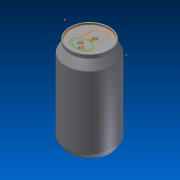
# Autodesk Inventor part: cocacola can
Saved by Autodesk Inventor 2019 (Build 230136000, 136)
## iProperties
Created: 2011-12-12
Part Number: cocacola can
Material: Generic
Document SubType Name: Modeling
Designer: roedger3
Density: 1 g/cm^3
Appearance: Default
Author: roedger3
Autodesk Inventor part; units mm, degrees
ref_plane "YZ Plane" through (0, 0, 0) normal (1, 0, 0) x (0, 1, 0)
ref_plane "XZ Plane" through (0, 0, 0) normal (0, 1, 0) x (-1, 0, 0)
ref_plane "XY Plane" through (0, 0, 0) normal (0, 0, 1) x (1, 0, 0)
sketch "Sketch1" plane through (0, 0, 0) normal (0, 0, 1) x (1, 0, 0)
  line L0 (-5.0988, -3.9037) -> (-5.0988, -101.0858)
  line L1 (0.463, -109.3372) -> (-0.635, -109.3372)
  line L2 (1.0329, 8.8525) -> (1.0329, 10.9702)
  line L3 (0.6383, 7.3196) -> (-4.7042, -2.3707)
  line L4 (-0.635, -109.3372) -> (-0.635, -109.3228)
  line L5 (-1.2355, -107.4647) -> (-4.4983, -102.9439)
  arc A0 (-5.0988, -101.0858) -> (-4.4983, -102.9439) centre (-1.9238, -101.0858) ccw
  arc A1 (-0.635, -109.3228) -> (-1.2355, -107.4647) centre (-3.81, -109.3228) ccw
  arc A2 (-4.7042, -2.3707) -> (-5.0988, -3.9037) centre (-1.9238, -3.9037) ccw
  arc A3 (0.6383, 7.3196) -> (1.0329, 8.8525) centre (-2.1421, 8.8525) ccw
  line L6 (1.0329, 10.9702) -> (0.6426, 10.9702)
  line L7 (0.3886, 11.2242) -> (0.3886, 13.0908)
  line L8 (0.6426, 13.3448) -> (1.5362, 13.3448)
  line L9 (1.7902, 13.0908) -> (1.7902, 11.2242)
  line L10 (2.0442, 10.9702) -> (27.7942, 10.9702)
  arc A4 (0.3886, 11.2242) -> (0.6426, 10.9702) centre (0.6426, 11.2242) ccw
  arc A5 (0.6426, 13.3448) -> (0.3886, 13.0908) centre (0.6426, 13.0908) ccw
  arc A6 (1.7902, 13.0908) -> (1.5362, 13.3448) centre (1.5362, 13.0908) ccw
  arc A7 (1.7902, 11.2242) -> (2.0442, 10.9702) centre (2.0442, 11.2242) ccw
  line L11 (27.7942, 10.9702) -> (27.7942, -95.2167)
  ellipse E0 centre (27.7942, 0) end of major axis (-3.3972, 0) minor radius 9.4787 (27.7942, 9.4787) -> (2.7229, 5.6391) ccw
  arc A8 (2.7229, 5.6391) -> (-4.9986, -3.1122) centre (11.6697, -10.0371) ccw
  arc A9 (27.7942, -95.2167) -> (3.1136, -106.0246) centre (27.585, -128.3229) ccw
  ellipse E1 centre (27.7942, -109.3372) end of major axis (27.7942, -101.6264) minor radius 27.3312 (27.7942, -101.6264) -> (0.463, -109.3372) ccw
  line L12 (27.7942, -95.2167) -> (27.7942, -101.6264)
  point P0 (0, 0)
  dimension "d8" = 3.175
  dimension "d20" = 0.254
  dimension "d21" = 122.682
  constraints: 26 end point, 21 point on circle, 15 tangent, 10 centre point, 6 equal radius, 4 perpendicular, 2 point on line, 2 vertical, 1 horizontal, 1 parallel, 9 other
  measures "d8" radius of A0
  measures "d20" radius of A4
  measures "d21" distance from line of L1 L8.start
revolve "Revolution1" add sketch "Sketch1" angle 360 about axis through (27.7942, 10.9702, 0) along (0, -1, 0) contours A2 A8 L3 E0 L11 A9 E1 L1 L4 A1 L5 A0 L0 | A2 L3 A8 | L3 A3 L2 L6 A4 L7 A5 L8 A6 L9 A7 L10 L11 E0 A8
sketch "Sketch3" plane through (27.7942, 10.9702, 0) normal (0, 1, 0) x (1, 0, 0)
  circle A0 centre (0, 0) radius 25.75 projected
  point P0 (-27.7942, 0)
sketch "Sketch4" plane through (27.7942, 10.9702, 0) normal (0, 1, 0) x (1, 0, 0)
  ellipse E0 centre (-0.043, -10.033) end of major axis (-11.981, -10.033) minor radius 8.255
  point P0 (-27.7942, 0)
  dimension "d23" = 11.938
  dimension "d24" = 8.255
  constraints: 2 other
sketch "Sketch5" plane through (27.7942, 10.9702, 0) normal (0, 1, 0) x (1, 0, 0)
  circle A0 centre (0, 0) radius 25.75 projected
  point P0 (-27.7942, 0)
shell "Shell1" [suppressed]
sketch "Sketch6" plane through (27.7942, 10.9702, 0) normal (0, 1, 0) x (1, 0, 0)
  ellipse E0 centre (-0.043, -10.033) end of major axis (11.895, -10.033) minor radius 8.255 projected
  circle A0 centre (0, 0) radius 25.75 projected
  ellipse E1 centre (-0.043, -10.033) end of major axis (-0.043, 0) minor radius 13.716 (-11.748, -4.803) -> (11.6621, -4.803) ccw
  arc A1 (9.3327, 9.75) -> (-9.3977, 9.637) centre (-0.043, 11.4301) ccw
  line L0 (0, 0) -> (0, 1.9052)
  arc A2 (-11.748, -4.803) -> (-9.568, 11.4301) centre (-41.662, 7.4773) ccw
  arc A3 (9.482, 11.4301) -> (11.6621, -4.803) centre (42.7111, 7.6297) ccw
  point P0 (-27.7942, 0)
  dimension "d8" = 3.175
  dimension "d33" = 13.716
  dimension "d34" = 10.033
  constraints: 11 point on circle, 3 centre point, 2 end point, 1 coincident, 1 vertical, 5 other
extrude "Extrusion2" cut sketch "Sketch6" against normal blind 0.254 contours A2 A1 A3 E1
sketch "Sketch7" plane through (27.7942, 10.7162, 0) normal (0, 1, 0) x (1, 0, 0)
  circle A0 centre (0, 0) radius 1.905
  point P0 (11.895, -10.033)
  point P1 (-27.7942, 0)
  dimension "d42" = 3.81
  constraints: 1 centre point
  measures "d42" diameter of A0
extrude "Extrusion3" add sketch "Sketch7" along normal blind 0.635
sketch "Sketch8" plane through (27.7942, 10.7162, 0) normal (0, 1, 0) x (1, 0, 0)
  arc A0 (0.647, -1.7918) -> (-0.6551, -1.7888) centre (0, 0) ccw projected
  ellipse E0 centre (-0.043, -10.033) end of major axis (-11.981, -10.033) minor radius 8.255 (-0.6551, -1.7888) -> (0.647, -1.7918) ccw projected
  arc A1 (9.482, 11.4301) -> (11.6621, -4.803) centre (42.7111, 7.6297) ccw projected
  arc A2 (9.482, 11.4301) -> (-9.568, 11.4301) centre (-0.043, 11.4301) ccw projected
  arc A3 (-11.748, -4.803) -> (-9.568, 11.4301) centre (-41.662, 7.4773) ccw projected
  ellipse E1 centre (-0.043, -10.033) end of major axis (-13.759, -10.033) minor radius 10.033 (-11.748, -4.803) -> (11.6621, -4.803) ccw projected
  arc A4 (1.7205, -1.8685) -> (-1.729, -1.8607) centre (0, 0) ccw
  point P0 (-27.7942, 0)
  dimension "d45" = 5.08
  constraints: 2 point on circle, 1 centre point, 1 coincident, 4 other
  measures "d45" diameter of A4
chamfer "Chamfer2" distance 0.254 angle 45 4 edges at (27.7512, 10.9702, 20.066) (18.181, 10.9702, -3.1733) (27.7512, 10.9702, -20.9551) (37.3572, 10.9702, -3.1781)
sketch "Sketch9" plane through (27.7942, 11.3512, 0) normal (0, 1, 0) x (1, 0, 0)
  circle A0 centre (0, 0) radius 1.905 projected
  point P0 (-27.7942, 0)
body "Solid1"
